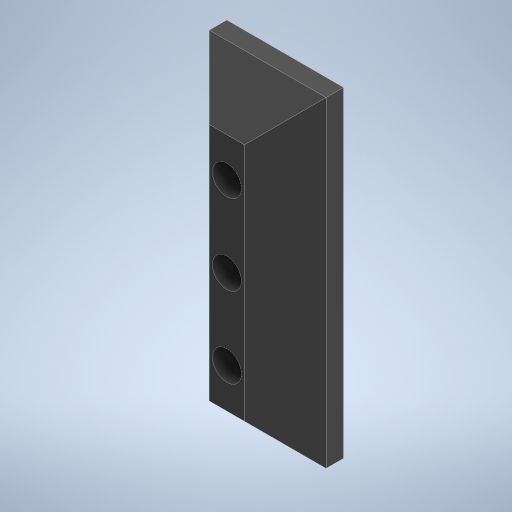
# Autodesk Inventor part: shield
Saved by Autodesk Inventor 2024.1 (Build 281209000, 209)
## iProperties
Created: 2024-02-14
Part Number: shield
Material: 一般
Document SubType Name: Modeling
Designer: hibik
Density: 1 g/cm^3
Appearance: 既定
Author: hibik
Autodesk Inventor part; units mm, degrees
ref_plane "YZ Plane" through (0, 0, 0) normal (1, 0, 0) x (0, 1, 0)
ref_plane "XZ Plane" through (0, 0, 0) normal (0, 1, 0) x (-1, 0, 0)
ref_plane "XY Plane" through (0, 0, 0) normal (0, 0, 1) x (1, 0, 0)
sketch "スケッチ1" plane through (0, 0, 0) normal (0, 0, 1) x (1, 0, 0)
  line L0 (0, 55) -> (20, 55)
  line L1 (20, 55) -> (20, 0)
  line L2 (20, 0) -> (0, 0)
  line L3 (0, 0) -> (0, 55)
  dimension "d0" = 20
  dimension "d1" = 55
  constraints: 8 end point, 2 parallel, 1 coincident, 1 horizontal, 1 perpendicular
  measures "d0" distance of L0.start L0.end
  measures "d1" distance of L2.end L0.start
extrude "押し出し1" add sketch "スケッチ1" along normal blind 10
chamfer "面取り1" distance 7 angle 45 4 edges at (20, 27.5, 10) (0, 27.5, 10) (10, 55, 10) (10, 0, 10)
sketch "スケッチ2" plane through (0, 0, 0) normal (0, 0, -1) x (-1, 0, 0)
  line L0 (0, 0) -> (-20, 0) projected
  line L1 (0, 55) -> (0, 0) projected
  line L2 (-20, 55) -> (0, 55) projected
  line L3 (-20, 0) -> (-20, 55) projected
  circle A0 centre (-10, 41.25) radius 0.8
  circle A1 centre (-10, 13.75) radius 0.8
  circle A2 centre (-10, 27.5) radius 0.8
  point P0 (-10, 55)
  dimension "d7" = 1.6
  dimension "d8" = 1.6
  dimension "d9" = 1.6
  dimension "d10" = 13.75
  dimension "d11" = 13.75
  dimension "d12" = 13.75
  dimension "d13" = 13.75
  constraints: 3 centre point, 3 vertical alignment, 1 midpoint
  measures "d7" diameter of A0
  measures "d8" diameter of A1
  measures "d9" diameter of A2
  measures "d10" distance from line of L2 A0.centre
  measures "d11" distance of A2.centre A0.centre
  measures "d12" distance of A1.centre A2.centre
  measures "d13" distance from line of L0 A1.centre
extrude "押し出し2" cut sketch "スケッチ2" against normal through all contours A0 | A1 | A2
sketch "スケッチ3" plane through (0, 0, 10) normal (0, 0, 1) x (1, 0, 0)
  circle A0 centre (10, 41.25) radius 0.8 projected
  circle A1 centre (10, 27.5) radius 0.8 projected
  circle A2 centre (10, 13.75) radius 0.8 projected
  circle A3 centre (10, 27.5) radius 0.8 projected
  circle A4 centre (10, 41.25) radius 0.8 projected
  line L0 (7, 7) -> (7, 48) projected
  line L1 (13, 7) -> (7, 7) projected
  line L2 (13, 48) -> (13, 7) projected
  line L3 (7, 48) -> (13, 48) projected
  circle A5 centre (10, 41.25) radius 2.5
  circle A6 centre (10, 27.5) radius 2.5
  circle A7 centre (10, 13.75) radius 2.5
  point P0 (0, 0)
  dimension "d16" = 5
  dimension "d17" = 5
  dimension "d18" = 5
  constraints: 3 centre point, 3 coincident
  measures "d16" diameter of A5
  measures "d17" diameter of A6
  measures "d18" diameter of A7
extrude "押し出し3" cut sketch "スケッチ3" against normal blind 8.5 contours A5 | A6 | A7
equation "\"d10\" = d13"
equation "\"d11\" = d13"
equation "\"d12\" = d13"
